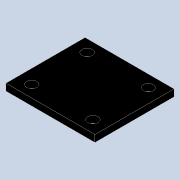
# Autodesk Inventor part: X Axis Belt Adjustable Top
Saved by Autodesk Inventor 2022 (Build 260153000, 153)
## iProperties
Created: 2021-10-20
Part Number: X Axis Belt Adjustable Top
Material: Generic
Document SubType Name: Modeling
Designer: Coy
Density: 1 g/cm^3
Appearance: Anodized - Black
Author: Coy
Autodesk Inventor part; units mm, degrees
ref_plane "YZ Plane" through (0, 0, 0) normal (1, 0, 0) x (0, 1, 0)
ref_plane "XZ Plane" through (0, 0, 0) normal (0, 1, 0) x (-1, 0, 0)
ref_plane "XY Plane" through (0, 0, 0) normal (0, 0, 1) x (1, 0, 0)
sketch "Sketch1" plane through (0, 0, 0) normal (0, 1, 0) x (-1, 0, 0)
  line L0 (17.2372, 12) -> (17.2372, 28) construction
  line L1 (14.9628, 12) -> (17.2372, 12) construction
  line L2 (14.9628, 12) -> (14.9628, 28) construction
  line L3 (17.2372, 28) -> (14.9628, 28) construction
  line L4 (14.2372, 12) -> (14.2372, 28) construction
  line L5 (11.9628, 12) -> (14.2372, 12) construction
  line L6 (11.9628, 12) -> (11.9628, 28) construction
  line L7 (14.2372, 28) -> (11.9628, 28) construction
  line L8 (20.2372, 28) -> (17.9628, 28) construction
  line L9 (20.2372, 12) -> (20.2372, 28) construction
  line L10 (17.9628, 12) -> (20.2372, 12) construction
  line L11 (17.9628, 12) -> (17.9628, 28) construction
  line L12 (11.2372, 12) -> (11.2372, 28) construction
  line L13 (8.9628, 12) -> (11.2372, 12) construction
  line L14 (8.9628, 12) -> (8.9628, 28) construction
  line L15 (11.2372, 28) -> (8.9628, 28) construction
  line L16 (23.2372, 28) -> (20.9628, 28) construction
  line L17 (23.2372, 12) -> (23.2372, 28) construction
  line L18 (20.9628, 12) -> (23.2372, 12) construction
  line L19 (20.9628, 12) -> (20.9628, 28) construction
  line L20 (8.2372, 12) -> (8.2372, 28) construction
  line L21 (5.9628, 12) -> (8.2372, 12) construction
  line L22 (5.9628, 12) -> (5.9628, 28) construction
  line L23 (8.2372, 28) -> (5.9628, 28) construction
  line L24 (26.2372, 28) -> (23.9628, 28) construction
  line L25 (26.2372, 12) -> (26.2372, 28) construction
  line L26 (23.9628, 12) -> (26.2372, 12) construction
  line L27 (23.9628, 12) -> (23.9628, 28) construction
  line L28 (5.2372, 12) -> (5.2372, 28) construction
  line L29 (2.9628, 12) -> (5.2372, 12) construction
  line L30 (2.9628, 12) -> (2.9628, 28) construction
  line L31 (5.2372, 28) -> (2.9628, 28) construction
  line L32 (29.2372, 28) -> (26.9628, 28) construction
  line L33 (29.2372, 12) -> (29.2372, 28) construction
  line L34 (26.9628, 12) -> (29.2372, 12) construction
  line L35 (26.9628, 12) -> (26.9628, 28) construction
  line L36 (2.2372, 12) -> (2.2372, 28) construction
  line L37 (0, 12) -> (2.2372, 12) construction
  line L38 (0, 0) -> (0, 28)
  line L39 (45, 0) -> (0, 0)
  line L40 (45, 28) -> (45, 0)
  line L41 (43.8628, 12) -> (45, 12) construction
  line L42 (43.8628, 12) -> (43.8628, 28) construction
  line L43 (45, 28) -> (43.8628, 28) construction
  line L44 (45, 40) -> (45, 28)
  line L45 (0, 40) -> (45, 40)
  line L46 (0, 28) -> (0, 40)
  line L47 (2.2372, 28) -> (0, 28) construction
  circle A0 centre (7.05, 34) radius 2.6
  circle A1 centre (37.95, 34) radius 2.6
  circle A2 centre (37.95, 6) radius 2.6
  circle A3 centre (7.05, 6) radius 2.6
  line L48 (32.2372, 28) -> (29.9628, 28) construction
  line L49 (32.2372, 12) -> (32.2372, 28) construction
  line L50 (29.9628, 12) -> (32.2372, 12) construction
  line L51 (29.9628, 12) -> (29.9628, 28) construction
  line L52 (37.95, 6) -> (7.05, 6) construction
  line L53 (7.05, 6) -> (7.05, 34) construction
  line L54 (7.05, 34) -> (37.95, 34) construction
  line L55 (37.95, 34) -> (37.95, 6) construction
  point P0 (34.1, 12)
  dimension "d2" = 45
  dimension "d3" = 40
  dimension "d4" = 30.9
  constraints: 112 end point, 4 centre point, 2 parallel, 2 point on line, 1 coincident, 1 horizontal, 1 perpendicular
  measures "d2" distance of L39.start L38.start
  measures "d3" distance of L45.start point (0, 0)
  measures "d4" distance of L52.start L52.end
extrude "Extrusion1" add sketch "Sketch1" along normal blind 3.5
body "Solid1"
